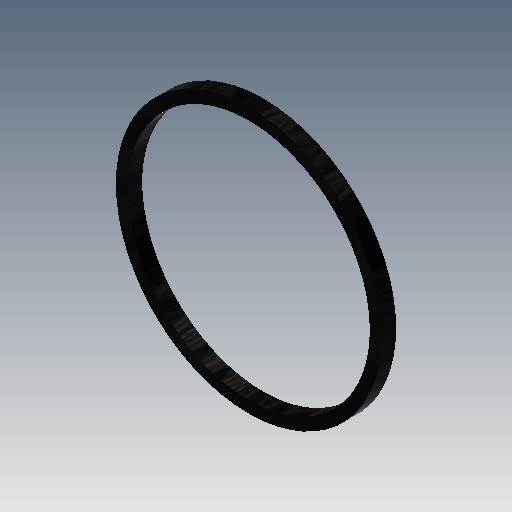
# Autodesk Inventor part: 軸受け用ワッシャD_ダブルスラスト用(t3_ジュラコン)
Saved by Autodesk Inventor 2019.4 (Build 234330000, 330)
## iProperties
Created: 2018-08-10
Part Number: 軸受け用ワッシャD_ダブルスラスト用(t3_ジュラコン)
Material: アセタール樹脂、黒
Document SubType Name: Modeling
Designer: Owner
Density: 1.425 g/cm^3
Appearance: 滑らか - 黒
Mass: 0.971459 g
Surface Area: 12.2711 cm^2
Volume: 0.681726 cm^3
Author: Owner
Autodesk Inventor part; units mm, degrees
ref_plane "YZ Plane" through (0, 0, 0) normal (1, 0, 0) x (0, 1, 0)
ref_plane "XZ Plane" through (0, 0, 0) normal (0, 1, 0) x (-1, 0, 0)
ref_plane "XY Plane" through (0, 0, 0) normal (0, 0, 1) x (1, 0, 0)
sketch "スケッチ1" plane through (0, 0, 0) normal (0, 0, 1) x (1, 0, 0)
  circle A0 centre (0, 0) radius 20.7
  circle A1 centre (0, 0) radius 22.7
  dimension "d0" = 41.4
  dimension "d1" = 45.4
  constraints: 2 centre point, 2 coincident
  measures "d0" diameter of A0
  measures "d1" diameter of A1
extrude "押し出し1" add sketch "スケッチ1" along normal blind 2.5
